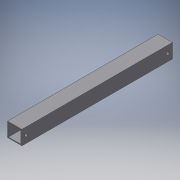
# Autodesk Inventor part: push bar
Saved by Autodesk Inventor 2018 (Build 220112000, 112)
## iProperties
Created: 2019-01-18
Part Number: push bar
Material: Generic
Document SubType Name: Modeling
Designer: s-4008082
Density: 1 g/cm^3
Appearance: Default
Mass: 61.8401 g
Surface Area: 492.386 cm^2
Volume: 61.8401 cm^3
Author: s-4008082
Autodesk Inventor part; units mm, degrees
ref_plane "YZ Plane" through (0, 0, 0) normal (1, 0, 0) x (0, 1, 0)
ref_plane "XZ Plane" through (0, 0, 0) normal (0, 1, 0) x (-1, 0, 0)
ref_plane "XY Plane" through (0, 0, 0) normal (0, 0, 1) x (1, 0, 0)
sketch "Sketch1" plane through (0, 0, 0) normal (0, 0, 1) x (1, 0, 0)
  line L0 (12.7, -12.7) -> (-12.7, -12.7)
  line L1 (-12.7, -12.7) -> (-12.7, 12.7)
  line L2 (-12.7, 12.7) -> (12.7, 12.7)
  line L3 (12.7, 12.7) -> (12.7, -12.7)
  line L4 (12.7, -12.7) -> (-12.7, 12.7) construction
  line L5 (-12.7, -12.7) -> (12.7, 12.7) construction
  line L6 (11.049, 11.049) -> (-11.049, 11.049)
  line L7 (-11.049, 11.049) -> (-11.049, -11.049)
  line L8 (-11.049, -11.049) -> (11.049, -11.049)
  line L9 (11.049, -11.049) -> (11.049, 11.049)
  line L10 (11.049, 11.049) -> (-11.049, -11.049) construction
  line L11 (-11.049, 11.049) -> (11.049, -11.049) construction
  point P0 (0, 0)
  dimension "d0" = 25.4
  dimension "d1" = 25.4
  dimension "d2" = 1.651
  dimension "d3" = 1.651
  constraints: 24 end point, 4 midpoint, 4 parallel, 2 horizontal, 2 perpendicular
  measures "d0" distance of L1.end L2.end
  measures "d1" distance of L0.end L1.end
  measures "d2" distance between parallel lines of L1 L7
  measures "d3" distance between parallel lines of L0 L8
extrude "Extrusion1" add sketch "Sketch1" along normal blind 266.7
sketch "Sketch2" plane through (12.7, -12.7, 0) normal (1, 0, 0) x (0, 0, -1)
  circle A0 centre (-8.1788, 12.7) radius 2.54
  circle A1 centre (-259.08, 12.7) radius 2.54
  line L0 (0, 25.4) -> (0, 0) projected
  line L1 (-266.7, 0) -> (-266.7, 25.4) projected
  line L2 (0, 0) -> (-266.7, 0) projected
  point P0 (0, 12.7)
  dimension "d6" = 250.9012
  dimension "d7" = 5.08
  dimension "d8" = 5.08
  dimension "d15" = 12.7
  dimension "d16" = 12.7
  dimension "d17" = 7.62
  constraints: 2 centre point
  measures "d6" distance of A0.centre A1.centre
  measures "d7" diameter of A0
  measures "d8" diameter of A1
  measures "d15" distance from line of L2 A0.centre
  measures "d16" distance from line of L2 A1.centre
  measures "d17" distance from line of L1 A1.centre
extrude "Extrusion2" cut sketch "Sketch2" against normal blind 2.54
equation "\"d3\" = d2"
equation "\"d8\" = d7"
body "Solid1"
